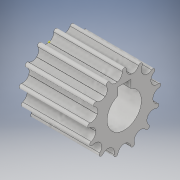
# Autodesk Inventor part: MotorGear
Saved by Autodesk Inventor 2018 (Build 220112000, 112)
## iProperties
Created: 2019-06-11
Part Number: MotorGear
Material: Generic
Document SubType Name: Modeling
Designer: anirudh
Density: 1 g/cm^3
Appearance: Default
Author: anirudh
Autodesk Inventor part; units mm, degrees
ref_plane "YZ Plane" through (0, 0, 0) normal (1, 0, 0) x (0, 1, 0)
ref_plane "XZ Plane" through (0, 0, 0) normal (0, 1, 0) x (-1, 0, 0)
ref_plane "XY Plane" through (0, 0, 0) normal (0, 0, 1) x (1, 0, 0)
sketch "Sketch1" plane through (0, 0, 0) normal (1, 0, 0) x (0, 1, 0)
  arc A0 (3.7081, 1.5) -> (3.7081, -1.5) centre (0, 0) ccw
  arc A1 (6.5427, 1.6009) -> (8.0964, 0.4688) centre (7.99, 1.955) ccw
  arc A2 (8.0964, -0.4688) -> (6.5427, -1.6009) centre (7.99, -1.955) ccw
  arc A3 (8.0964, -0.4688) -> (8.0964, 0.4688) centre (8.13, 0) ccw
  arc A4 (5.0493, 4.458) -> (6.9512, 4.1777) centre (6.1663, 5.4442) ccw
  arc A5 (7.3869, 3.3475) -> (6.9512, 4.1777) centre (7.1988, 3.7782) ccw
  arc A6 (7.3869, 3.3475) -> (6.5372, 1.623) centre (7.9833, 1.9821) ccw
  arc A7 (2.3992, 6.2939) -> (4.2135, 6.9295) centre (2.9299, 7.6862) ccw
  arc A8 (4.9851, 6.3969) -> (4.2135, 6.9295) centre (4.6184, 6.6909) ccw
  arc A9 (4.9851, 6.3969) -> (5.0342, 4.4751) centre (6.1478, 5.4651) ccw
  arc A10 (-0.8006, 6.688) -> (0.5105, 8.0939) centre (-0.9777, 8.1674) ccw
  arc A11 (1.4413, 7.9809) -> (0.5105, 8.0939) centre (0.98, 8.0707) ccw
  arc A12 (1.4413, 7.9809) -> (2.3778, 6.302) centre (2.9038, 7.6961) ccw
  arc A13 (-3.8169, 5.5498) -> (-3.3094, 7.4041) centre (-4.6612, 6.7775) ccw
  arc A14 (-2.4327, 7.7365) -> (-3.3094, 7.4041) centre (-2.8829, 7.6017) ccw
  arc A15 (-2.4327, 7.7365) -> (-0.8232, 6.6852) centre (-1.0053, 8.164) ccw
  arc A16 (-5.9589, 3.1403) -> (-6.3711, 5.018) centre (-7.277, 3.835) ccw
  arc A17 (-5.7494, 5.7198) -> (-6.3711, 5.018) centre (-6.0854, 5.3912) ccw
  arc A18 (-5.7494, 5.7198) -> (-3.8357, 5.5369) centre (-4.6842, 6.7617) ccw
  arc A19 (-6.7357, 0.0114) -> (-7.9734, 1.4824) centre (-8.2257, 0.0139) ccw
  arc A20 (-7.749, 2.3928) -> (-7.9734, 1.4824) centre (-7.8938, 1.9456) ccw
  arc A21 (-7.749, 2.3928) -> (-5.9695, 3.1201) centre (-7.29, 3.8103) ccw
  arc A22 (-5.9695, -3.1201) -> (-7.749, -2.3928) centre (-7.29, -3.8103) ccw
  arc A23 (-7.9734, -1.4824) -> (-7.749, -2.3928) centre (-7.8938, -1.9456) ccw
  arc A24 (-7.9734, -1.4824) -> (-6.7357, -0.0114) centre (-8.2257, -0.0139) ccw
  arc A25 (-3.8357, -5.5369) -> (-5.7494, -5.7198) centre (-4.6842, -6.7617) ccw
  arc A26 (-6.3711, -5.018) -> (-5.7494, -5.7198) centre (-6.0854, -5.3912) ccw
  arc A27 (-6.3711, -5.018) -> (-5.9589, -3.1403) centre (-7.277, -3.835) ccw
  arc A28 (-0.8232, -6.6852) -> (-2.4327, -7.7365) centre (-1.0053, -8.164) ccw
  arc A29 (-3.3094, -7.4041) -> (-2.4327, -7.7365) centre (-2.8829, -7.6017) ccw
  arc A30 (-3.3094, -7.4041) -> (-3.8169, -5.5498) centre (-4.6612, -6.7775) ccw
  arc A31 (2.3778, -6.302) -> (1.4413, -7.9809) centre (2.9038, -7.6961) ccw
  arc A32 (0.5105, -8.0939) -> (1.4413, -7.9809) centre (0.98, -8.0707) ccw
  arc A33 (0.5105, -8.0939) -> (-0.8006, -6.688) centre (-0.9777, -8.1674) ccw
  arc A34 (5.0342, -4.4751) -> (4.9851, -6.3969) centre (6.1478, -5.4651) ccw
  arc A35 (4.2135, -6.9295) -> (4.9851, -6.3969) centre (4.6184, -6.6909) ccw
  arc A36 (4.2135, -6.9295) -> (2.3992, -6.2939) centre (2.9299, -7.6862) ccw
  arc A37 (6.5372, -1.623) -> (7.3869, -3.3475) centre (7.9833, -1.9821) ccw
  arc A38 (6.9512, -4.1777) -> (7.3869, -3.3475) centre (7.1988, -3.7782) ccw
  arc A39 (6.9512, -4.1777) -> (5.0493, -4.458) centre (6.1663, -5.4442) ccw
  arc A40 (6.5427, 1.6009) -> (6.5372, 1.623) centre (0, 0) ccw
  arc A41 (6.5372, -1.623) -> (6.5427, -1.6009) centre (0, 0) ccw
  arc A42 (5.0493, 4.458) -> (5.0342, 4.4751) centre (0, 0) ccw
  arc A43 (2.3992, 6.2939) -> (2.3778, 6.302) centre (0, 0) ccw
  arc A44 (-0.8006, 6.688) -> (-0.8232, 6.6852) centre (0, 0) ccw
  arc A45 (-3.8169, 5.5498) -> (-3.8357, 5.5369) centre (0, 0) ccw
  arc A46 (-5.9589, 3.1403) -> (-5.9695, 3.1201) centre (0, 0) ccw
  arc A47 (-6.7357, 0.0114) -> (-6.7357, -0.0114) centre (0, 0) ccw
  arc A48 (-5.9695, -3.1201) -> (-5.9589, -3.1403) centre (0, 0) ccw
  arc A49 (-3.8357, -5.5369) -> (-3.8169, -5.5498) centre (0, 0) ccw
  arc A50 (-0.8232, -6.6852) -> (-0.8006, -6.688) centre (0, 0) ccw
  arc A51 (2.3778, -6.302) -> (2.3992, -6.2939) centre (0, 0) ccw
  arc A52 (5.0342, -4.4751) -> (5.0493, -4.458) centre (0, 0) ccw
  line L0 (5.5, 0) -> (5.5, 1.5)
  line L1 (5.5, 1.5) -> (3.7081, 1.5)
  line L2 (3.7081, -1.5) -> (5.5, -1.5)
  line L3 (5.5, -1.5) -> (5.5, 0)
  dimension "d13" = 360
  constraints: 109 point on circle, 53 centre point, 8 end point, 2 coincident, 1 perpendicular, 1 tangent, 1 vertical, 131 other
extrude "Extrusion2" add sketch "Sketch1" along normal blind 16
body "Solid2"
